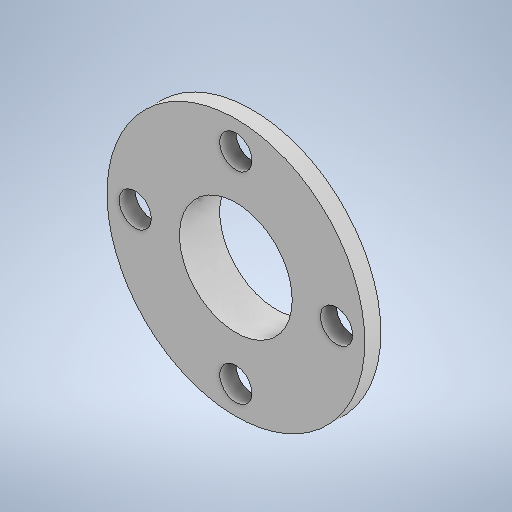
# Autodesk Inventor part: flange
Saved by Autodesk Inventor 2025 (Build 290162000, 162)
## iProperties
Created: 2025-01-08
Part Number: flange
Material: Generic
Document SubType Name: Modeling
Designer: 5014070
Density: 1 g/cm^3
Appearance: Default
Author: 5014070
Autodesk Inventor part; units mm, degrees
ref_plane "YZ Plane" through (0, 0, 0) normal (1, 0, 0) x (0, 1, 0)
ref_plane "XZ Plane" through (0, 0, 0) normal (0, 1, 0) x (-1, 0, 0)
ref_plane "XY Plane" through (0, 0, 0) normal (0, 0, 1) x (1, 0, 0)
sketch "Sketch1" plane through (0, 0, 0) normal (0, 0, 1) x (1, 0, 0)
  circle A0 centre (0, 0) radius 7
  circle A1 centre (0, 0) radius 16
  circle A2 centre (-12.5, 0) radius 2
  circle A3 centre (0, -12.5) radius 2
  circle A4 centre (12.5, 0) radius 2
  circle A5 centre (0, 12.5) radius 2
  circle A6 centre (0, 0) radius 8
  line L0 (0, 0) -> (-12.5, 0)
  point P0 (-7, 0)
  point P1 (-7.7857, 1.8392)
  dimension "d0" = 14
  dimension "d8" = 16
  dimension "d1" = 32
  dimension "d2" = 4
  dimension "d5" = 360
  dimension "d15" = 12.5
  constraints: 5 centre point, 4 coincident, 2 end point, 1 horizontal alignment, 14 other
  measures "d1" diameter of A1
  measures "d2" diameter of A2
  measures "d15" distance of L0.start L0.end
extrude "Extrusion1" add sketch "Sketch1" along normal blind 2 contours A1
extrude "Extrusion2" add sketch "Sketch1" against normal blind 3 contours A6
extrude "Extrusion3" add sketch "Sketch1" along normal blind 2 contours A6
fillet "Fillet2" radius 0.5 1 edges at (-8, 0, 0)
body "Solid1"
